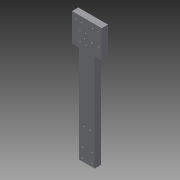
# Autodesk Inventor part: Arm-SquareBar-Rev3
Saved by Autodesk Inventor 2015 (Build 190159000, 159)
## iProperties
Created: 2017-01-08
Part Number: Arm-SquareBar-Rev3
Material: Generic
Document SubType Name: Modeling
Designer: Guy
Density: 1 g/cm^3
Appearance: Default
Mass: 295.484 g
Surface Area: 443.772 cm^2
Volume: 295.484 cm^3
Author: Guy
Autodesk Inventor part; units mm, degrees
ref_plane "YZ Plane" through (0, 0, 0) normal (1, 0, 0) x (0, 1, 0)
ref_plane "XZ Plane" through (0, 0, 0) normal (0, 1, 0) x (-1, 0, 0)
ref_plane "XY Plane" through (0, 0, 0) normal (0, 0, 1) x (1, 0, 0)
sketch "Sketch1" plane through (0, 0, 0) normal (0, 0, 1) x (1, 0, 0)
  line L0 (0, 0) -> (95, 0)
  line L1 (95, 0) -> (95, 20)
  line L2 (95, 20) -> (0, 20)
  line L3 (0, 20) -> (0, 0)
  dimension "d0" = 95
  dimension "d1" = 20
  constraints: 8 end point, 2 parallel, 1 horizontal, 1 perpendicular
  measures "d0" distance of L1.end L2.end
  measures "d1" distance of L0.end L1.end
extrude "Extrusion1" add sketch "Sketch1" along normal blind 400
sketch "Sketch4" plane through (0, 20, 0) normal (0, 1, 0) x (1, 0, 0)
  line L0 (95, 0) -> (0, 0) projected
  line L1 (0, 0) -> (0, -400) projected
  line L2 (95, -400) -> (0, -400) projected
  line L3 (95, 0) -> (95, -400) projected
  line L4 (95, -376.825) -> (95, -383.175) projected
  line L5 (0, -383.175) -> (0, -376.825) projected
  line L6 (95, 0) -> (72.5, 0)
  line L7 (72.5, 0) -> (72.5, -310)
  line L8 (72.5, -310) -> (95, -310)
  line L9 (95, -310) -> (95, 0)
  line L10 (0, 0) -> (22.5, 0)
  line L11 (22.5, 0) -> (22.5, -310)
  line L12 (22.5, -310) -> (0, -310)
  line L13 (0, -310) -> (0, 0)
  dimension "d30" = 90
  dimension "d31" = 50
  dimension "d32" = 22.5
  constraints: 16 end point, 4 parallel, 2 horizontal, 2 perpendicular, 1 point on line
  measures "d30" distance between parallel lines of L12 L2
  measures "d31" distance between parallel lines of L7 L11
  measures "d32" distance between parallel lines of L3 L7
extrude "Extrusion4" cut sketch "Sketch4" against normal up to next contours L3 L8 L7 L0 | L11 L12 L1 L0
sketch "Sketch5" plane through (0, 20, 400) normal (0, 1, 0) x (1, 0, 0)
  circle A0 centre (62.5, 360) radius 2.5
  circle A1 centre (32.5, 360) radius 2.5
  circle A2 centre (62.5, 390) radius 2.5
  circle A3 centre (32.5, 390) radius 2.5
  line L0 (22.5, 400) -> (22.5, 90) projected
  line L1 (22.5, 90) -> (0, 90) projected
  line L2 (0, 90) -> (0, 0) projected
  line L3 (95, 0) -> (0, 0) projected
  line L4 (95, 90) -> (95, 0) projected
  line L5 (95, 90) -> (72.5, 90) projected
  line L6 (72.5, 90) -> (72.5, 400) projected
  line L7 (72.5, 400) -> (22.5, 400) projected
  point P0 (0, 400)
  dimension "d35" = 5
  dimension "d36" = 5
  dimension "d37" = 5
  dimension "d38" = 5
  dimension "d39" = 30
  dimension "d40" = 30
  dimension "d41" = 10
  dimension "d42" = 10
  dimension "d43" = 30
  dimension "d44" = 30
  dimension "d45" = 10
  dimension "d46" = 10
  constraints: 4 centre point
  measures "d35" diameter of A2
  measures "d36" diameter of A3
  measures "d37" diameter of A1
  measures "d38" diameter of A0
  measures "d39" distance of A1.centre A0.centre
  measures "d40" distance of A3.centre A2.centre
  measures "d41" distance from line of L6 A0.centre
  measures "d42" distance from line of L6 A2.centre
  measures "d43" distance of A2.centre A0.centre
  measures "d44" distance of A3.centre A1.centre
  measures "d45" distance from line of L7 A3.centre
  measures "d46" distance from line of L7 A2.centre
extrude "Extrusion5" cut sketch "Sketch5" against normal up to next contours A0 | A1 | A2 | A3
sketch "Sketch8" plane through (0, 20, 400) normal (0, 1, 0) x (1, 0, 0)
  circle A0 centre (30.325, 15) radius 2.425
  circle A1 centre (11.925, 15) radius 2.425
  circle A2 centre (83.075, 15) radius 2.425
  circle A3 centre (64.675, 15) radius 2.425
  line L0 (0, 90) -> (0, 0) projected
  line L1 (95, 90) -> (95, 0) projected
  line L2 (95, 0) -> (0, 0) projected
  point P0 (0, 400)
  dimension "d60" = 4.85
  dimension "d61" = 4.85
  dimension "d62" = 4.85
  dimension "d63" = 4.85
  dimension "d64" = 11.925
  dimension "d65" = 18.4
  dimension "d66" = 11.925
  dimension "d67" = 18.4
  dimension "d68" = 15
  dimension "d69" = 15
  dimension "d70" = 15
  dimension "d71" = 15
  constraints: 4 centre point
  measures "d60" diameter of A1
  measures "d61" diameter of A0
  measures "d62" diameter of A3
  measures "d63" diameter of A2
  measures "d64" distance from line of L0 A1.centre
  measures "d65" distance of A0.centre A1.centre
  measures "d66" distance from line of L1 A2.centre
  measures "d67" distance of A2.centre A3.centre
  measures "d68" distance from line of A2.centre L2
  measures "d69" distance from line of A3.centre L2
  measures "d70" distance from line of L2 A0.centre
  measures "d71" distance from line of L2 A1.centre
extrude "Extrusion8" cut sketch "Sketch8" against normal up to next
sketch "Sketch9" plane through (0, 20, 400) normal (0, 1, 0) x (1, 0, 0)
  circle A0 centre (43.5, 40) radius 2.15
  circle A1 centre (43.5, 71.8) radius 2.15
  line L0 (95, 0) -> (0, 0) projected
  line L1 (0, 90) -> (0, 0) projected
  circle A2 centre (24.5, 40) radius 2.15
  circle A3 centre (24.5, 71.8) radius 2.15
  point P0 (0, 400)
  dimension "d74" = 4.3
  dimension "d75" = 4.3
  dimension "d76" = 31.8
  dimension "d77" = 40
  dimension "d80" = 4.3
  dimension "d81" = 4.3
  dimension "d82" = 19
  dimension "d83" = 19
  dimension "d84" = 31.8
  dimension "d85" = 40
  dimension "d86" = 24.5
  dimension "d87" = 24.5
  constraints: 4 centre point
  measures "d74" diameter of A0
  measures "d75" diameter of A1
  measures "d76" distance of A1.centre A0.centre
  measures "d77" distance from line of A0.centre L0
  measures "d80" diameter of A2
  measures "d81" diameter of A3
  measures "d82" distance of A0.centre A2.centre
  measures "d83" distance of A1.centre A3.centre
  measures "d84" distance of A3.centre A2.centre
  measures "d85" distance from line of L0 A2.centre
  measures "d86" distance from line of L1 A2.centre
  measures "d87" distance from line of L1 A3.centre
extrude "Extrusion9" cut sketch "Sketch9" against normal up to next
sketch "Sketch10" plane through (0, 20, 400) normal (0, 1, 0) x (1, 0, 0)
  circle A0 centre (84.5, 55.9) radius 2.5
  circle A1 centre (39.5, 55.9) radius 2.5
  circle A2 centre (24.5, 40) radius 2.15 projected
  circle A3 centre (43.5, 40) radius 2.15 projected
  circle A4 centre (43.5, 71.8) radius 2.15 projected
  circle A5 centre (24.5, 71.8) radius 2.15 projected
  circle A6 centre (83.075, 15) radius 2.425 projected
  circle A7 centre (30.325, 15) radius 2.425 projected
  circle A8 centre (11.925, 15) radius 2.425 projected
  circle A9 centre (64.675, 15) radius 2.425 projected
  circle A10 centre (62.5, 390) radius 2.5 projected
  circle A11 centre (62.5, 360) radius 2.5 projected
  circle A12 centre (32.5, 360) radius 2.5 projected
  circle A13 centre (32.5, 390) radius 2.5 projected
  line L0 (22.5, 400) -> (22.5, 90) projected
  line L1 (22.5, 90) -> (0, 90) projected
  line L2 (0, 90) -> (0, 0) projected
  line L3 (95, 0) -> (0, 0) projected
  line L4 (95, 90) -> (95, 0) projected
  line L5 (95, 90) -> (72.5, 90) projected
  line L6 (72.5, 90) -> (72.5, 400) projected
  line L7 (72.5, 400) -> (22.5, 400) projected
  circle A14 centre (62, 55.9) radius 3.175
  point P0 (0, 400)
  dimension "d90" = 45
  dimension "d91" = 5
  dimension "d92" = 5
  dimension "d93" = 15.9
  dimension "d94" = 15.9
  dimension "d95" = 39.5
  dimension "d106" = 6.35
  dimension "d107" = 22.5
  dimension "d108" = 15.9
  constraints: 3 centre point
  measures "d90" distance of A0.centre A1.centre
  measures "d91" diameter of A1
  measures "d92" diameter of A0
  measures "d93" vertical distance of A1.centre A3.centre
  measures "d94" vertical distance of A0.centre A3.centre
  measures "d95" distance from line of L2 A1.centre
  measures "d106" diameter of A14
  measures "d107" distance of A14.centre A1.centre
  measures "d108" vertical distance of A14.centre A3.centre
extrude "Extrusion10" cut sketch "Sketch10" against normal up to next contours A0 | A1 | A14
sketch "Sketch11" plane through (0, 20, 400) normal (0, 1, 0) x (1, 0, 0)
  circle A0 centre (57.5, 300) radius 2.5
  circle A1 centre (37.5, 300) radius 2.5
  line L0 (72.5, 400) -> (22.5, 400) projected
  line L1 (72.5, 90) -> (72.5, 400) projected
  point P0 (0, 400)
  dimension "d98" = 5
  dimension "d99" = 5
  dimension "d100" = 20
  dimension "d101" = 100
  dimension "d102" = 100
  dimension "d103" = 15
  constraints: 2 centre point
  measures "d98" diameter of A0
  measures "d99" diameter of A1
  measures "d100" distance of A1.centre A0.centre
  measures "d101" distance from line of L0 A1.centre
  measures "d102" distance from line of L0 A0.centre
  measures "d103" distance from line of L1 A0.centre
extrude "Extrusion11" cut sketch "Sketch11" against normal up to next
equation "\"d87\" = d86"
body "Solid1"
